Autodesk Fusion 360 part; units mm, degrees
(part 4 of 4)
  line L248 (168.6977, -94.525) -> (158.6977, -94.525)
  arc A252 (158.6977, -91.525) -> (158.6977, -94.525) centre (158.6977, -93.025) ccw
  line L249 (158.6977, -91.525) -> (168.6977, -91.525)
  arc A253 (248.6977, -114.525) -> (248.6977, -111.525) centre (248.6977, -113.025) ccw
  line L250 (248.6977, -114.525) -> (238.6977, -114.525)
  arc A254 (238.6977, -111.525) -> (238.6977, -114.525) centre (238.6977, -113.025) ccw
  line L251 (238.6977, -111.525) -> (248.6977, -111.525)
  arc A255 (168.6977, -54.525) -> (168.6977, -51.525) centre (168.6977, -53.025) ccw
  line L252 (168.6977, -54.525) -> (158.6977, -54.525)
  arc A256 (158.6977, -51.525) -> (158.6977, -54.525) centre (158.6977, -53.025) ccw
  line L253 (158.6977, -51.525) -> (168.6977, -51.525)
  arc A257 (168.6977, -74.525) -> (168.6977, -71.525) centre (168.6977, -73.025) ccw
  line L254 (168.6977, -74.525) -> (158.6977, -74.525)
  arc A258 (158.6977, -71.525) -> (158.6977, -74.525) centre (158.6977, -73.025) ccw
  line L255 (158.6977, -71.525) -> (168.6977, -71.525)
  arc A259 (248.6977, -104.525) -> (248.6977, -101.525) centre (248.6977, -103.025) ccw
  line L256 (248.6977, -104.525) -> (238.6977, -104.525)
  arc A260 (238.6977, -101.525) -> (238.6977, -104.525) centre (238.6977, -103.025) ccw
  line L257 (238.6977, -101.525) -> (248.6977, -101.525)
  arc A261 (228.6977, -164.525) -> (228.6977, -161.525) centre (228.6977, -163.025) ccw
  line L258 (228.6977, -164.525) -> (218.6977, -164.525)
  arc A262 (218.6977, -161.525) -> (218.6977, -164.525) centre (218.6977, -163.025) ccw
  line L259 (218.6977, -161.525) -> (228.6977, -161.525)
  arc A263 (208.6977, -164.525) -> (208.6977, -161.525) centre (208.6977, -163.025) ccw
  line L260 (208.6977, -164.525) -> (198.6977, -164.525)
  arc A264 (198.6977, -161.525) -> (198.6977, -164.525) centre (198.6977, -163.025) ccw
  line L261 (198.6977, -161.525) -> (208.6977, -161.525)
  arc A265 (188.6977, -144.525) -> (188.6977, -141.525) centre (188.6977, -143.025) ccw
  line L262 (188.6977, -144.525) -> (178.6977, -144.525)
  arc A266 (178.6977, -141.525) -> (178.6977, -144.525) centre (178.6977, -143.025) ccw
  line L263 (178.6977, -141.525) -> (188.6977, -141.525)
  arc A267 (188.6977, 35.475) -> (188.6977, 38.475) centre (188.6977, 36.975) ccw
  line L264 (188.6977, 35.475) -> (178.6977, 35.475)
  arc A268 (178.6977, 38.475) -> (178.6977, 35.475) centre (178.6977, 36.975) ccw
  line L265 (178.6977, 38.475) -> (188.6977, 38.475)
  arc A269 (188.6977, -54.525) -> (188.6977, -51.525) centre (188.6977, -53.025) ccw
  line L266 (188.6977, -54.525) -> (178.6977, -54.525)
  arc A270 (178.6977, -51.525) -> (178.6977, -54.525) centre (178.6977, -53.025) ccw
  line L267 (178.6977, -51.525) -> (188.6977, -51.525)
  arc A271 (128.6977, -134.525) -> (128.6977, -131.525) centre (128.6977, -133.025) ccw
  line L268 (128.6977, -134.525) -> (118.6977, -134.525)
  arc A272 (118.6977, -131.525) -> (118.6977, -134.525) centre (118.6977, -133.025) ccw
  line L269 (118.6977, -131.525) -> (128.6977, -131.525)
  arc A273 (88.6977, -84.525) -> (88.6977, -81.525) centre (88.6977, -83.025) ccw
  line L270 (88.6977, -84.525) -> (78.6977, -84.525)
  arc A274 (78.6977, -81.525) -> (78.6977, -84.525) centre (78.6977, -83.025) ccw
  line L271 (78.6977, -81.525) -> (88.6977, -81.525)
  arc A275 (188.6977, -84.525) -> (188.6977, -81.525) centre (188.6977, -83.025) ccw
  line L272 (188.6977, -84.525) -> (178.6977, -84.525)
  arc A276 (178.6977, -81.525) -> (178.6977, -84.525) centre (178.6977, -83.025) ccw
  line L273 (178.6977, -81.525) -> (188.6977, -81.525)
  arc A277 (188.6977, 15.475) -> (188.6977, 18.475) centre (188.6977, 16.975) ccw
  line L274 (188.6977, 15.475) -> (178.6977, 15.475)
  arc A278 (178.6977, 18.475) -> (178.6977, 15.475) centre (178.6977, 16.975) ccw
  line L275 (178.6977, 18.475) -> (188.6977, 18.475)
  arc A279 (128.6977, -114.525) -> (128.6977, -111.525) centre (128.6977, -113.025) ccw
  line L276 (128.6977, -114.525) -> (118.6977, -114.525)
  arc A280 (118.6977, -111.525) -> (118.6977, -114.525) centre (118.6977, -113.025) ccw
  line L277 (118.6977, -111.525) -> (128.6977, -111.525)
  arc A281 (248.6977, -84.525) -> (248.6977, -81.525) centre (248.6977, -83.025) ccw
  line L278 (248.6977, -84.525) -> (238.6977, -84.525)
  arc A282 (238.6977, -81.525) -> (238.6977, -84.525) centre (238.6977, -83.025) ccw
  line L279 (238.6977, -81.525) -> (248.6977, -81.525)
  arc A283 (88.6977, -104.525) -> (88.6977, -101.525) centre (88.6977, -103.025) ccw
  line L280 (88.6977, -104.525) -> (78.6977, -104.525)
  arc A284 (78.6977, -101.525) -> (78.6977, -104.525) centre (78.6977, -103.025) ccw
  line L281 (78.6977, -101.525) -> (88.6977, -101.525)
  arc A285 (128.6977, -154.525) -> (128.6977, -151.525) centre (128.6977, -153.025) ccw
  line L282 (128.6977, -154.525) -> (118.6977, -154.525)
  arc A286 (118.6977, -151.525) -> (118.6977, -154.525) centre (118.6977, -153.025) ccw
  line L283 (118.6977, -151.525) -> (128.6977, -151.525)
  arc A287 (228.6977, -104.525) -> (228.6977, -101.525) centre (228.6977, -103.025) ccw
  line L284 (228.6977, -104.525) -> (218.6977, -104.525)
  arc A288 (218.6977, -101.525) -> (218.6977, -104.525) centre (218.6977, -103.025) ccw
  line L285 (218.6977, -101.525) -> (228.6977, -101.525)
  arc A289 (188.6977, -134.525) -> (188.6977, -131.525) centre (188.6977, -133.025) ccw
  line L286 (188.6977, -134.525) -> (178.6977, -134.525)
  arc A290 (178.6977, -131.525) -> (178.6977, -134.525) centre (178.6977, -133.025) ccw
  line L287 (178.6977, -131.525) -> (188.6977, -131.525)
  arc A291 (228.6977, -74.525) -> (228.6977, -71.525) centre (228.6977, -73.025) ccw
  line L288 (228.6977, -74.525) -> (218.6977, -74.525)
  arc A292 (218.6977, -71.525) -> (218.6977, -74.525) centre (218.6977, -73.025) ccw
  line L289 (218.6977, -71.525) -> (228.6977, -71.525)
  arc A293 (188.6977, -104.525) -> (188.6977, -101.525) centre (188.6977, -103.025) ccw
  line L290 (188.6977, -104.525) -> (178.6977, -104.525)
  arc A294 (178.6977, -101.525) -> (178.6977, -104.525) centre (178.6977, -103.025) ccw
  line L291 (178.6977, -101.525) -> (188.6977, -101.525)
  arc A295 (208.6977, -124.525) -> (208.6977, -121.525) centre (208.6977, -123.025) ccw
  line L292 (208.6977, -124.525) -> (198.6977, -124.525)
  arc A296 (198.6977, -121.525) -> (198.6977, -124.525) centre (198.6977, -123.025) ccw
  line L293 (198.6977, -121.525) -> (208.6977, -121.525)
  arc A297 (68.6977, -84.525) -> (68.6977, -81.525) centre (68.6977, -83.025) ccw
  line L294 (68.6977, -84.525) -> (58.6977, -84.525)
  arc A298 (58.6977, -81.525) -> (58.6977, -84.525) centre (58.6977, -83.025) ccw
  line L295 (58.6977, -81.525) -> (68.6977, -81.525)
  arc A299 (148.6977, -54.525) -> (148.6977, -51.525) centre (148.6977, -53.025) ccw
  line L296 (148.6977, -54.525) -> (138.6977, -54.525)
  arc A300 (138.6977, -51.525) -> (138.6977, -54.525) centre (138.6977, -53.025) ccw
  line L297 (138.6977, -51.525) -> (148.6977, -51.525)
  arc A301 (248.6977, -94.525) -> (248.6977, -91.525) centre (248.6977, -93.025) ccw
  line L298 (248.6977, -94.525) -> (238.6977, -94.525)
  arc A302 (238.6977, -91.525) -> (238.6977, -94.525) centre (238.6977, -93.025) ccw
  line L299 (238.6977, -91.525) -> (248.6977, -91.525)
  arc A303 (208.6977, -184.525) -> (208.6977, -181.525) centre (208.6977, -183.025) ccw
  line L300 (208.6977, -184.525) -> (198.6977, -184.525)
  arc A304 (198.6977, -181.525) -> (198.6977, -184.525) centre (198.6977, -183.025) ccw
  line L301 (198.6977, -181.525) -> (208.6977, -181.525)
  arc A305 (108.6977, -94.525) -> (108.6977, -91.525) centre (108.6977, -93.025) ccw
  line L302 (108.6977, -94.525) -> (98.6977, -94.525)
  arc A306 (98.6977, -91.525) -> (98.6977, -94.525) centre (98.6977, -93.025) ccw
  line L303 (98.6977, -91.525) -> (108.6977, -91.525)
  arc A307 (128.6977, -14.525) -> (128.6977, -11.525) centre (128.6977, -13.025) ccw
  line L304 (128.6977, -14.525) -> (118.6977, -14.525)
  arc A308 (118.6977, -11.525) -> (118.6977, -14.525) centre (118.6977, -13.025) ccw
  line L305 (118.6977, -11.525) -> (128.6977, -11.525)
  arc A309 (188.6977, -94.525) -> (188.6977, -91.525) centre (188.6977, -93.025) ccw
  line L306 (188.6977, -94.525) -> (178.6977, -94.525)
  arc A310 (178.6977, -91.525) -> (178.6977, -94.525) centre (178.6977, -93.025) ccw
  line L307 (178.6977, -91.525) -> (188.6977, -91.525)
  arc A311 (168.6977, -134.525) -> (168.6977, -131.525) centre (168.6977, -133.025) ccw
  line L308 (168.6977, -134.525) -> (158.6977, -134.525)
  arc A312 (158.6977, -131.525) -> (158.6977, -134.525) centre (158.6977, -133.025) ccw
  line L309 (158.6977, -131.525) -> (168.6977, -131.525)
  arc A313 (128.6977, -144.525) -> (128.6977, -141.525) centre (128.6977, -143.025) ccw
  line L310 (128.6977, -144.525) -> (118.6977, -144.525)
  arc A314 (118.6977, -141.525) -> (118.6977, -144.525) centre (118.6977, -143.025) ccw
  line L311 (118.6977, -141.525) -> (128.6977, -141.525)
  arc A315 (88.6977, -74.525) -> (88.6977, -71.525) centre (88.6977, -73.025) ccw
  line L312 (88.6977, -74.525) -> (78.6977, -74.525)
  arc A316 (78.6977, -71.525) -> (78.6977, -74.525) centre (78.6977, -73.025) ccw
  line L313 (78.6977, -71.525) -> (88.6977, -71.525)
  arc A317 (148.6977, -84.525) -> (148.6977, -81.525) centre (148.6977, -83.025) ccw
  line L314 (148.6977, -84.525) -> (138.6977, -84.525)
  arc A318 (138.6977, -81.525) -> (138.6977, -84.525) centre (138.6977, -83.025) ccw
  line L315 (138.6977, -81.525) -> (148.6977, -81.525)
  arc A319 (108.6977, -104.525) -> (108.6977, -101.525) centre (108.6977, -103.025) ccw
  line L316 (108.6977, -104.525) -> (98.6977, -104.525)
  arc A320 (98.6977, -101.525) -> (98.6977, -104.525) centre (98.6977, -103.025) ccw
  line L317 (98.6977, -101.525) -> (108.6977, -101.525)
  arc A321 (168.6977, -84.525) -> (168.6977, -81.525) centre (168.6977, -83.025) ccw
  line L318 (168.6977, -84.525) -> (158.6977, -84.525)
  arc A322 (158.6977, -81.525) -> (158.6977, -84.525) centre (158.6977, -83.025) ccw
  line L319 (158.6977, -81.525) -> (168.6977, -81.525)
  arc A323 (228.6977, -64.525) -> (228.6977, -61.525) centre (228.6977, -63.025) ccw
  line L320 (228.6977, -64.525) -> (218.6977, -64.525)
  arc A324 (218.6977, -61.525) -> (218.6977, -64.525) centre (218.6977, -63.025) ccw
  line L321 (218.6977, -61.525) -> (228.6977, -61.525)
  arc A325 (228.6977, -84.525) -> (228.6977, -81.525) centre (228.6977, -83.025) ccw
  line L322 (228.6977, -84.525) -> (218.6977, -84.525)
  arc A326 (218.6977, -81.525) -> (218.6977, -84.525) centre (218.6977, -83.025) ccw
  line L323 (218.6977, -81.525) -> (228.6977, -81.525)
  arc A327 (148.6977, -114.525) -> (148.6977, -111.525) centre (148.6977, -113.025) ccw
  line L324 (148.6977, -114.525) -> (138.6977, -114.525)
  arc A328 (138.6977, -111.525) -> (138.6977, -114.525) centre (138.6977, -113.025) ccw
  line L325 (138.6977, -111.525) -> (148.6977, -111.525)
  arc A329 (168.6977, -154.525) -> (168.6977, -151.525) centre (168.6977, -153.025) ccw
  line L326 (168.6977, -154.525) -> (158.6977, -154.525)
  arc A330 (158.6977, -151.525) -> (158.6977, -154.525) centre (158.6977, -153.025) ccw
  line L327 (158.6977, -151.525) -> (168.6977, -151.525)
  arc A331 (68.6977, -74.525) -> (68.6977, -71.525) centre (68.6977, -73.025) ccw
  line L328 (68.6977, -74.525) -> (58.6977, -74.525)
  arc A332 (58.6977, -71.525) -> (58.6977, -74.525) centre (58.6977, -73.025) ccw
  line L329 (58.6977, -71.525) -> (68.6977, -71.525)
  arc A333 (128.6977, -64.525) -> (128.6977, -61.525) centre (128.6977, -63.025) ccw
  line L330 (128.6977, -64.525) -> (118.6977, -64.525)
  arc A334 (118.6977, -61.525) -> (118.6977, -64.525) centre (118.6977, -63.025) ccw
  line L331 (118.6977, -61.525) -> (128.6977, -61.525)
  arc A335 (248.6977, -134.525) -> (248.6977, -131.525) centre (248.6977, -133.025) ccw
  line L332 (248.6977, -134.525) -> (238.6977, -134.525)
  arc A336 (238.6977, -131.525) -> (238.6977, -134.525) centre (238.6977, -133.025) ccw
  line L333 (238.6977, -131.525) -> (248.6977, -131.525)
  arc A337 (128.6977, -104.525) -> (128.6977, -101.525) centre (128.6977, -103.025) ccw
  line L334 (128.6977, -104.525) -> (118.6977, -104.525)
  arc A338 (118.6977, -101.525) -> (118.6977, -104.525) centre (118.6977, -103.025) ccw
  line L335 (118.6977, -101.525) -> (128.6977, -101.525)
  arc A339 (208.6977, -4.525) -> (208.6977, -1.525) centre (208.6977, -3.025) ccw
  line L336 (208.6977, -4.525) -> (198.6977, -4.525)
  arc A340 (198.6977, -1.525) -> (198.6977, -4.525) centre (198.6977, -3.025) ccw
  line L337 (198.6977, -1.525) -> (208.6977, -1.525)
  arc A341 (208.6977, -134.525) -> (208.6977, -131.525) centre (208.6977, -133.025) ccw
  line L338 (208.6977, -134.525) -> (198.6977, -134.525)
  arc A342 (198.6977, -131.525) -> (198.6977, -134.525) centre (198.6977, -133.025) ccw
  line L339 (198.6977, -131.525) -> (208.6977, -131.525)
  arc A343 (128.6977, -124.525) -> (128.6977, -121.525) centre (128.6977, -123.025) ccw
  line L340 (128.6977, -124.525) -> (118.6977, -124.525)
  arc A344 (118.6977, -121.525) -> (118.6977, -124.525) centre (118.6977, -123.025) ccw
  line L341 (118.6977, -121.525) -> (128.6977, -121.525)
  arc A345 (128.6977, -54.525) -> (128.6977, -51.525) centre (128.6977, -53.025) ccw
  line L342 (128.6977, -54.525) -> (118.6977, -54.525)
  arc A346 (118.6977, -51.525) -> (118.6977, -54.525) centre (118.6977, -53.025) ccw
  line L343 (118.6977, -51.525) -> (128.6977, -51.525)
  arc A347 (208.6977, -14.525) -> (208.6977, -11.525) centre (208.6977, -13.025) ccw
  line L344 (208.6977, -14.525) -> (198.6977, -14.525)
  arc A348 (198.6977, -11.525) -> (198.6977, -14.525) centre (198.6977, -13.025) ccw
  line L345 (198.6977, -11.525) -> (208.6977, -11.525)
  arc A349 (108.6977, -134.525) -> (108.6977, -131.525) centre (108.6977, -133.025) ccw
  line L346 (108.6977, -134.525) -> (98.6977, -134.525)
  arc A350 (98.6977, -131.525) -> (98.6977, -134.525) centre (98.6977, -133.025) ccw
  line L347 (98.6977, -131.525) -> (108.6977, -131.525)
  arc A351 (88.6977, -94.525) -> (88.6977, -91.525) centre (88.6977, -93.025) ccw
  line L348 (88.6977, -94.525) -> (78.6977, -94.525)
  arc A352 (78.6977, -91.525) -> (78.6977, -94.525) centre (78.6977, -93.025) ccw
  line L349 (78.6977, -91.525) -> (88.6977, -91.525)
  arc A353 (148.6977, -174.525) -> (148.6977, -171.525) centre (148.6977, -173.025) ccw
  line L350 (148.6977, -174.525) -> (138.6977, -174.525)
  arc A354 (138.6977, -171.525) -> (138.6977, -174.525) centre (138.6977, -173.025) ccw
  line L351 (138.6977, -171.525) -> (148.6977, -171.525)
  arc A355 (108.6977, -124.525) -> (108.6977, -121.525) centre (108.6977, -123.025) ccw
  line L352 (108.6977, -124.525) -> (98.6977, -124.525)
  arc A356 (98.6977, -121.525) -> (98.6977, -124.525) centre (98.6977, -123.025) ccw
  line L353 (98.6977, -121.525) -> (108.6977, -121.525)
component "Electronics Plate" placed x (1, 0, 0) y (0, 1, 0) z (0, 0, 1) at (0, 0, 0)
